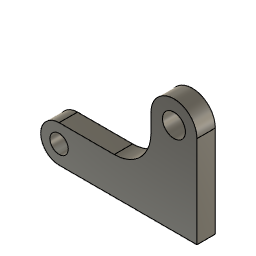
Part 7 (Autodesk Fusion 360 design; units mm, degrees)
Autodesk Fusion 360 part; units mm, degrees
sketch "Sketch1" plane through (0, 0, 0) normal (0, 1, 0) x (1, 0, 0)
  line L0 (24.3392, -13.8982) -> (-125.6608, -13.8982)
  arc A0 (-125.6608, -13.8982) -> (-125.6608, -53.8982) centre (-125.6608, -33.8982) ccw
  arc A1 (-14.3201, -29.8888) -> (-14.3202, -29.8887) centre (-14.3202, -29.8888) ccw
  line L1 (-14.3201, -29.8888) -> (-14.3201, -30.0005)
  arc A2 (-25.6608, -113.8982) -> (24.3392, -113.8982) centre (-0.6608, -113.8982) ccw
  line L2 (24.3392, -113.8982) -> (24.3392, -13.8982)
  line L3 (-125.6608, -53.8982) -> (-65.6608, -53.8982)
  arc A3 (-25.6608, -93.8982) -> (-65.6608, -53.8982) centre (-65.6608, -93.8982) ccw
  line L4 (-25.6608, -93.8982) -> (-25.6608, -113.8982)
  circle A4 centre (-0.6608, -113.8982) radius 12.5
  circle A5 centre (-125.6608, -33.8982) radius 10
  dimension "d1" = 100
  dimension "d2" = 150
  dimension "d3" = 20
  dimension "d4" = 25
  dimension "d5" = 40
  dimension "d6" = 25
  dimension "d7" = 20
  constraint horizontal L0
  constraint tangent L0 A0
  constraint tangent A1 L1
  constraint vertical L2
  constraint tangent A0 L3
  constraint horizontal L3
  constraint tangent L3 A3
  constraint vertical L4
  constraint tangent A2 L4
  constraint tangent A2 L2
  constraint tangent A3 L4
  constraint concentric A2 A4
  constraint concentric A0 A5
  measures "d1" distance of L0.start A2.end
  measures "d2" distance of L0.start L0.end
  measures "d3" radius of A0
  measures "d4" radius of A2
  measures "d5" radius of A3
  measures "d6" diameter of A4
  measures "d7" diameter of A5
sketch "Sketch2" plane through (0, 0, 0) normal (0, 1, 0) x (1, 0, 0)
  line L0 (25, 100) -> (-125, 100)
  arc A0 (-125, 100) -> (-125, 60) centre (-125, 80) ccw
  line L1 (-125, 60) -> (-25, 60)
  line L2 (-25, 60) -> (-25, 0)
  arc A1 (-25, 0) -> (25, 0) centre (0, 0) ccw
  line L3 (25, 0) -> (25, 100)
  circle A2 centre (0, 0) radius 12.5
  circle A3 centre (-125, 80) radius 10
  dimension "d10" = 150
  dimension "d11" = 100
  dimension "d12" = 25
  dimension "d13" = 20
  dimension "d14" = 25
  dimension "d15" = 20
  constraint horizontal L0
  constraint tangent L0 A0
  constraint tangent A0 L1
  constraint parallel L0 L1
  constraint perpendicular L1 L2
  constraint tangent L2 A1
  constraint tangent A1 L3
  constraint vertical L3
  constraint coincident A1.centre A2.centre
  constraint concentric A1 A2
  constraint concentric A0 A3
  measures "d10" distance of L0.start L0.end
  measures "d11" distance of L0.start A1.end
  measures "d12" radius of A1
  measures "d13" radius of A0
  measures "d14" diameter of A2
  measures "d15" diameter of A3
extrude "Extrude2" add sketch "Sketch2" along normal blind 20
fillet "Fillet1" radius 40 1 edges at (-25, 10, -60)
